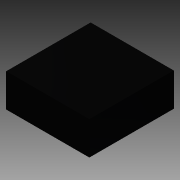
# Autodesk Inventor part: DRV
Saved by Autodesk Inventor 2015 SP1 (Build 190203100, 203)
## iProperties
Created: 2015-10-19
Part Number: DRV
Material: Generic
Document SubType Name: Modeling
Designer: Kartikye
Density: 1 g/cm^3
Appearance: DRV, DRV
Author: Kartikye
Autodesk Inventor part; units mm, degrees
ref_plane "YZ Plane" through (0, 0, 0) normal (1, 0, 0) x (0, 1, 0)
ref_plane "XZ Plane" through (0, 0, 0) normal (0, 1, 0) x (-1, 0, 0)
ref_plane "XY Plane" through (0, 0, 0) normal (0, 0, 1) x (1, 0, 0)
sketch "DRV, DRV_111" plane through (0, 0, 0) normal (0, 0, 1) x (1, 0, 0)
  line L0 (-0.8635, 0.1885) -> (1.65, 0.1885)
  line L1 (1.65, 0.1885) -> (1.65, -2.3635)
  line L2 (1.65, -2.3635) -> (-0.8635, -2.3635)
  line L3 (-0.8635, -2.3635) -> (-0.8635, 0.1885)
  constraints: 8 end point
extrude "Extrusion1" add sketch "DRV, DRV_111" along normal blind 1
body "Solid1"
